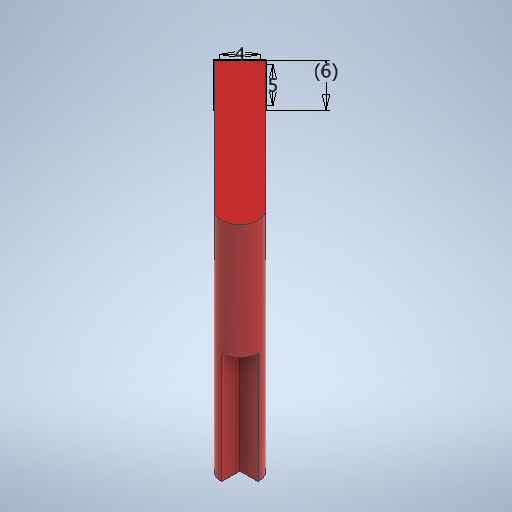
# Autodesk Inventor part: Redesign_Gripper_Finger
Saved by Autodesk Inventor 2025.1 (Build 291241000, 241)
## iProperties
Created: 2024-12-20
Part Number: Redesign_Gripper_Finger
Material: Generic
Document SubType Name: Modeling
Designer: m_kni
Density: 1 g/cm^3
Appearance: Default
Author: m_kni
Autodesk Inventor part; units mm, degrees
ref_plane "YZ Plane" through (0, 0, 0) normal (1, 0, 0) x (0, 1, 0)
ref_plane "XZ Plane" through (0, 0, 0) normal (0, 1, 0) x (-1, 0, 0)
ref_plane "XY Plane" through (0, 0, 0) normal (0, 0, 1) x (1, 0, 0)
sketch "Sketch1" plane through (0, 0, 0) normal (0, 1, 0) x (-1, 0, 0)
  arc A0 (-2.54, 0) -> (0, 2.54) centre (0, 0) ccw
  line L0 (0, 2.54) -> (0, 0)
  line L1 (0, 0) -> (-2.54, 0)
  dimension "d0" = 5.08
  constraints: 4 end point, 2 point on circle, 1 centre point, 1 coincident, 1 perpendicular, 1 vertical
  measures "d0" diameter of A0
extrude "Extrusion1" add sketch "Sketch1" along normal blind 25.4
sketch "Sketch2" plane through (0, 25.4, 0) normal (0, 1, 0) x (1, 0, 0)
  line L0 (0, -2.54) -> (0, 0) projected
  line L1 (0, 0) -> (-17.9605, 17.9605)
  line L2 (0, 0) -> (25.4, 0) construction
  line L3 (0, 0) -> (-1.7961, -1.7961)
  arc A0 (2.54, 0) -> (0, -2.54) centre (0, 0) ccw projected
  line L4 (0, 0) -> (1.7961, 1.7961)
  line L5 (-1.7961, -1.7961) -> (-19.7566, 16.1645)
  line L6 (-19.7566, 16.1645) -> (-17.9605, 17.9605)
  line L7 (-16.1645, 19.7566) -> (1.7961, 1.7961)
  line L8 (-16.1645, 19.7566) -> (-17.9605, 17.9605)
  line L9 (0, 0) -> (2.54, 0)
  dimension "d3" = 25.4
  dimension "d4" = 135
  constraints: 18 end point, 4 perpendicular, 3 point on circle, 2 horizontal, 2 point on line, 1 equal length, 1 tangent
  measures "d3" distance of L0.end L1.end
  measures "d4" angle of L2 L1
extrude "Extrusion2" add sketch "Sketch2" along normal blind 6
sketch "Sketch3" plane through (-19.7566, 25.4, -16.1645) normal (-0.7071068, 0, -0.7071068) x (-0.7071068, 0, 0.7071068)
  line L0 (-5.08, 0) -> (-5.08, 6) projected
  line L1 (0, 6) -> (-5.08, 6)
  line L2 (-5.08, 6) -> (-5.08, 0)
  line L3 (-5.08, 0) -> (0, 0)
  line L4 (0, 0.5) -> (0, 5.5)
  line L5 (-2.54, 6) -> (-4.3361, 6) projected
  line L6 (-2.54, 6) -> (-2.54, 0)
  line L7 (-4.54, 0) -> (-0.54, 0)
  line L8 (-0.54, 0.5) -> (-0.54, 5.5)
  line L9 (-0.54, 6) -> (-4.54, 6)
  line L10 (-4.54, 6) -> (-4.54, 0)
  line L11 (-4.54, 0) -> (-0.54, 6) construction
  line L12 (-0.54, 0) -> (-4.54, 6) construction
  line L13 (0, 0.5) -> (-5.08, 0.5)
  line L14 (-5.08, 0.5) -> (-5.08, 5.5)
  line L15 (-5.08, 5.5) -> (0, 5.5)
  line L16 (0, 0.5) -> (-5.08, 5.5) construction
  line L17 (-5.08, 0.5) -> (0, 5.5) construction
  line L18 (-5.08, 0) -> (0, 0)
  line L19 (0, 0) -> (0, 6)
  line L20 (0, 6) -> (-5.08, 6)
  line L21 (-5.08, 6) -> (-5.08, 0)
  line L22 (-5.08, 0) -> (0, 6) construction
  line L23 (0, 0) -> (-5.08, 6) construction
  line L24 (-0.7439, 6) -> (0, 6)
  line L25 (-5.08, 0) -> (0, 0)
  line L26 (0, 0) -> (0, 6)
  line L27 (0, 6) -> (-5.08, 6)
  line L28 (-5.08, 6) -> (-5.08, 0)
  line L29 (-5.08, 0) -> (0, 6) construction
  line L30 (0, 0) -> (-5.08, 6) construction
  line L31 (0, 6) -> (0, 0)
  point P0 (-2.54, -25.4)
  point P1 (-2.54, 3)
  point P2 (-4.54, 5.5)
  point P3 (-5.08, 5.5)
  point P4 (-5.08, 0.5)
  point P5 (-4.54, 0.5)
  dimension "d7" = 4
  dimension "d8" = 5
  dimension "d11" = 6
  constraints: 60 end point, 10 midpoint, 9 parallel, 5 horizontal, 5 perpendicular, 4 point on line, 1 collinear, 1 vertical
  measures "d7" distance of L9.end L9.start
  measures "d8" distance of L13.end L14.end
  measures "d11" distance of L0.start L1.end
sketch "Sketch5" plane through (0, 31.4, 0) normal (0, 1, 0) x (1, 0, 0)
  line L0 (0, 0) -> (2.54, 0) projected
  circle A0 centre (0, 0) radius 2.54
  constraints: 1 coincident, 1 horizontal alignment, 2 other
extrude "Extrusion4" add sketch "Sketch5" against normal blind 16
body "Solid1"
